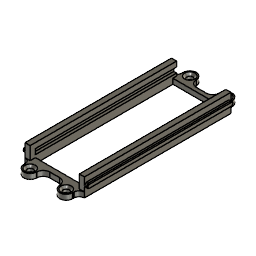
adapter (Autodesk Fusion 360 design; units mm, degrees)
Autodesk Fusion 360 part; units mm, degrees
note: some values were not read from the file. Set by a fixed rule: which face or edge a step refers to.
sketch "Sketch1" plane through (0, 0, 0) normal (1, 0, 0) x (0, 1, 0)
  line L0 (0, 0) -> (56.1898, 0)
  line L1 (56.1898, 0) -> (56.1898, 7)
  line L2 (56.1898, 7) -> (0, 7)
  line L3 (0, 7) -> (0, 0)
  dimension "d1" = 7
  constraint horizontal L0
  constraint vertical L1
  constraint horizontal L2
  constraint vertical L3
  constraint coincident L0.start L3.end
  measures "d1" distance of L0.start L2.end
extrude "Extrude1" add sketch "Sketch1" along normal blind 1
sketch "Sketch2" plane through (1, 0, 0) normal (1, 0, 0) x (0, 1, 0)
  line L0 (0, 7) -> (0, 0)
  line L1 (0, 0) -> (56.1898, 0)
  line L2 (56.1898, 0) -> (56.1898, 7)
  line L3 (56.1898, 7) -> (0, 7)
  line L4 (0, 0) -> (56.1898, 0)
  line L5 (56.1898, 0) -> (56.1898, 3)
  line L6 (56.1898, 3) -> (0, 3)
  line L7 (0, 3) -> (0, 0)
  line L8 (0, 7) -> (56.1898, 7)
  line L9 (56.1898, 7) -> (56.1898, 5)
  line L10 (56.1898, 5) -> (0, 5)
  line L11 (0, 5) -> (0, 7)
  line L12 (0, 3) -> (2, 3)
  line L13 (2, 3) -> (2, 5)
  line L14 (2, 5) -> (0, 5)
  line L15 (0, 5) -> (0, 3)
  dimension "d4" = 3
  dimension "d5" = 2
  dimension "d12" = 2
  constraint horizontal L4
  constraint vertical L5
  constraint horizontal L6
  constraint vertical L7
  constraint coincident L0.end L1.start
  constraint horizontal L8
  constraint vertical L9
  constraint horizontal L10
  constraint vertical L11
  constraint coincident L0.start L3.end
  constraint vertical L1.end L9.end
  constraint vertical L2.end L5.end
  constraint horizontal L12
  constraint vertical L13
  constraint horizontal L14
  constraint vertical L15
  measures "d4" distance of L0.end L6.end
  measures "d5" distance of L0.start L10.end
  measures "d12" distance of L6.end L12.end
extrude "Extrude2" add sketch "Sketch2" along normal blind 1 contours L0 L2 L3 L8 L9 L10 L11 L14 | L0 L6 L10 L12 L13 L14 L15 | L0 L1 L2 L4 L5 L6 L7 L12
sketch "Sketch3" plane through (0, 0, 0) normal (-1, 0, 0) x (0, -1, 0)
  line L0 (0, 0) -> (0, 7)
  line L1 (0, 7) -> (-56.1898, 7)
  line L2 (-56.1898, 7) -> (-56.1898, 0)
  line L3 (-56.1898, 0) -> (0, 0)
  line L4 (-56.1898, 3) -> (0, 3)
  line L5 (0, 3) -> (0, 4.9)
  line L6 (0, 4.9) -> (-56.1898, 4.9)
  line L7 (-56.1898, 4.9) -> (-56.1898, 3)
  dimension "d8" = 1.9
  dimension "d9" = 3
  constraint horizontal L4
  constraint vertical L5
  constraint horizontal L6
  constraint vertical L7
  constraint vertical L0.start L4.end
  constraint vertical L2.end L4.start
  measures "d8" distance of L4.start L6.end
  measures "d9" distance of L0.start L4.end
extrude "Extrude3" add sketch "Sketch3" along normal blind 1 contours L0 L2 L4 L5 L6 L7
sketch "Sketch4" plane through (2, 0, 0) normal (1, 0, 0) x (0, 1, 0)
  line L0 (0, 7) -> (0, 0)
  line L1 (0, 0) -> (56.1898, 0)
  line L2 (56.1898, 0) -> (56.1898, 3)
  line L3 (56.1898, 3) -> (2, 3)
  line L4 (2, 3) -> (2, 5)
  line L5 (2, 5) -> (56.1898, 5)
  line L6 (56.1898, 5) -> (56.1898, 7)
  line L7 (56.1898, 7) -> (0, 7)
  line L8 (0, 0) -> (2, 0)
  line L9 (2, 0) -> (2, 2)
  line L10 (2, 2) -> (0, 2)
  line L11 (0, 2) -> (0, 0)
  line L12 (56.1898, 0) -> (54.6898, 0)
  line L13 (54.6898, 0) -> (54.6898, 2)
  line L14 (54.6898, 2) -> (56.1898, 2)
  line L15 (56.1898, 2) -> (56.1898, 0)
  dimension "d13" = 2
  dimension "d14" = 2
  dimension "d15" = 1.5
  dimension "d16" = 2
  constraint horizontal L8
  constraint vertical L9
  constraint horizontal L10
  constraint vertical L11
  constraint coincident L0.end L1.start
  constraint horizontal L12
  constraint vertical L13
  constraint horizontal L14
  constraint vertical L15
  constraint coincident L1.end L2.start
  measures "d13" distance of L0.end L8.end
  measures "d14" distance of L0.end L10.end
  measures "d15" distance of L1.end L12.end
  measures "d16" distance of L1.end L14.end
extrude "Extrude4" add sketch "Sketch4" along normal blind 9.4 contours L0 L1 L8 L9 L10 L11 | L1 L2 L12 L13 L14 L15
mirror "Mirror1" about plane through (11.4, 0, 0) normal (1, 0, 0) of bodies 1 merged
extrude "Extrude5" cut 1 faces at (21.8, 20.0633, 4.3333) along direction (1, 0, 0) blind 0.1
extrude "Extrude6" cut 1 faces at (1, 20.0633, 4.3333) along direction (-1, 0, 0) blind 0.1
sketch "Sketch5" plane through (0, 0, 0) normal (0, 0, -1) x (1, 0, 0)
  line L0 (20.8, -54.6898) -> (2, -54.6898)
  line L1 (2, -54.6898) -> (2, -2)
  line L2 (2, -2) -> (20.8, -2)
  line L3 (20.8, -2) -> (20.8, -54.6898)
  line L4 (0, -56.1898) -> (22.8, -56.1898)
  line L5 (22.8, -56.1898) -> (22.8, 0)
  line L6 (22.8, 0) -> (0, 0)
  line L7 (0, 0) -> (0, -56.1898)
  line L8 (2, 0) -> (7, 0)
  line L9 (7, 0) -> (7, 5)
  line L10 (7, 5) -> (2, 5)
  line L11 (2, 5) -> (2, 0)
  line L12 (15.8, 0) -> (20.8, 0)
  line L13 (20.8, 0) -> (20.8, 5)
  line L14 (20.8, 5) -> (15.8, 5)
  line L15 (15.8, 5) -> (15.8, 0)
  line L16 (2, -56.1898) -> (7, -56.1898)
  line L17 (7, -56.1898) -> (7, -61.1898)
  line L18 (7, -61.1898) -> (2, -61.1898)
  line L19 (2, -61.1898) -> (2, -56.1898)
  line L20 (15.8, -56.1898) -> (20.8, -56.1898)
  line L21 (20.8, -56.1898) -> (20.8, -61.1898)
  line L22 (20.8, -61.1898) -> (15.8, -61.1898)
  line L23 (15.8, -61.1898) -> (15.8, -56.1898)
  dimension "d25" = 5
  dimension "d26" = 5
  dimension "d27" = 5
  dimension "d28" = 5
  dimension "d30" = 2
  dimension "d31" = 2
  dimension "d32" = 5
  dimension "d33" = 5
  dimension "d34" = 5
  dimension "d35" = 5
  dimension "d36" = 2
  dimension "d37" = 2
  constraint horizontal L8
  constraint vertical L9
  constraint horizontal L10
  constraint vertical L11
  constraint coincident L6 L8.start
  constraint horizontal L12
  constraint vertical L13
  constraint horizontal L14
  constraint vertical L15
  constraint horizontal L8.end L12.start
  constraint horizontal L16
  constraint vertical L17
  constraint horizontal L18
  constraint vertical L19
  constraint coincident L4 L16.start
  constraint horizontal L20
  constraint vertical L21
  constraint horizontal L22
  constraint vertical L23
  constraint coincident L4 L20.start
  measures "d25" distance of L8.start L8.end
  measures "d26" distance of L8.start L10.end
  measures "d27" distance of L12.start L12.end
  measures "d28" distance of L12.start L14.end
  measures "d30" distance of L7 L11
  measures "d31" distance of L5 L13
  measures "d32" distance of L16.start L16.end
  measures "d33" distance of L16.start L18.end
  measures "d34" distance of L20.start L20.end
  measures "d35" distance of L20.start L22.end
  measures "d36" distance of L7 L19
  measures "d37" distance of L5 L21
extrude "Extrude7" add sketch "Sketch5" against normal blind 2 contours L4 L16 L17 L18 L19 | L6 L8 L9 L10 L11 | L4 L20 L21 L22 L23 | L6 L12 L13 L14 L15
sketch "Sketch6" plane through (0, 0, 2) normal (0, 0, 1) x (-1, 0, 0)
  line L0 (-2, -2) -> (-2, 0)
  line L1 (-2, 0) -> (-2, 5)
  line L2 (-2, 5) -> (-7, 5)
  line L3 (-7, 5) -> (-7, 0)
  line L4 (-7, 0) -> (-15.8, 0)
  line L5 (-15.8, 0) -> (-15.8, 5)
  line L6 (-15.8, 5) -> (-20.8, 5)
  line L7 (-20.8, 5) -> (-20.8, 0)
  line L8 (-20.8, 0) -> (-20.8, -2)
  line L9 (-20.8, -2) -> (-2, -2)
  circle A0 centre (-4.5, 2.5) radius 0.5
  circle A1 centre (-18.3, 2.5) radius 0.5
  circle A2 centre (-4.5, -58.6898) radius 0.5
  circle A3 centre (-18.3, -58.6898) radius 0.5
  line L10 (-7, -61.1898) -> (-2, -61.1898)
  dimension "d40" = 1
  dimension "d41" = 1
  dimension "d42" = 1
  dimension "d43" = 1
  dimension "d44" = 2.5
  dimension "d45" = 2.5
  dimension "d46" = 2.5
  dimension "d47" = 2.5
  constraint horizontal A2.centre A3.centre
  constraint horizontal A0.centre A1.centre
  constraint vertical A1.centre A3.centre
  constraint vertical A0.centre A2.centre
  measures "d40" diameter of A0
  measures "d41" diameter of A1
  measures "d42" diameter of A2
  measures "d43" diameter of A3
  measures "d44" distance of A2.centre L10
  measures "d45" distance of L2 A0.centre
  measures "d46" distance of L3 A0.centre
  measures "d47" distance of L7 A1.centre
hole "Hole1" at (4.5, 58.6898, 2) at (18.3, 58.6898, 2) at (4.5, -2.5, 2) at (18.3, -2.5, 2) direction (0, 0, -1) diameter 2.3 depth 17 tip angle 180 countersink diameter 4 countersink angle 90
fillet "Fillet1" radius 2.5 12 edges at (7, -5, 1) (7, 0, 1) (2, -5, 1) (15.8, -5, 1) (20.8, -5, 1) (15.8, 0, 1) (20.8, 61.1898, 1) (15.8, 61.1898, 1) (7, 56.1898, 1) (7, 61.1898, 1) (2, 61.1898, 1) (15.8, 56.1898, 1)
fillet "Fillet1" radius 2 4 edges at (2, 56.1898, 1) (20.8, 56.1898, 1) (20.8, 0, 1) (2, 0, 1)
chamfer "Chamfer1" distance 0.8 angle 45 8 edges at (-0.5, 0, 4.9) (-0.5, 0, 3) (23.3, 0, 3) (23.3, 0, 4.9) (23.3, 56.1898, 4.9) (23.3, 56.1898, 3) (-0.5, 56.1898, 3) (-0.5, 56.1898, 4.9)
chamfer "Chamfer1" distance 0.3 angle 45 2 faces at (-1, 37.4599, 4.2667) (23.8, 37.4599, 4.2667)
equation "d17 = ( 20.8 / 2 ) * 1 mm - 1 mm"
